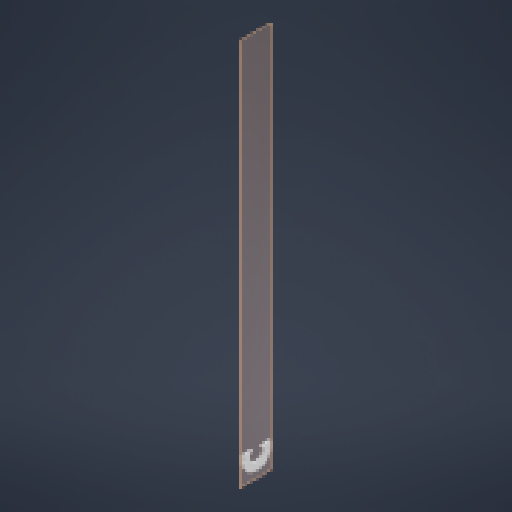
# Autodesk Inventor part: DropBarJoint
Saved by Autodesk Inventor 2024.1 (Build 281209000, 209)
## iProperties
Created: 2023-10-25
Part Number: DropBarJoint
Material: Generic
Document SubType Name: Modeling
Designer: Brandon
Density: 1 g/cm^3
Appearance: Default
Author: Brandon
Autodesk Inventor part; units mm, degrees
ref_plane "YZ Plane" through (0, 0, 0) normal (1, 0, 0) x (0, 1, 0)
ref_plane "XZ Plane" through (0, 0, 0) normal (0, 1, 0) x (-1, 0, 0)
ref_plane "XY Plane" through (0, 0, 0) normal (0, 0, 1) x (1, 0, 0)
ref_plane "Work Plane1" through (-214.9581, 261.0384, -210.6802) normal (1, 0, 0) x (0, 1, 0)
sketch "Sketch1" plane through (-214.9581, 261.0384, -210.6802) normal (1, 0, 0) x (0, 1, 0)
  arc A0 (-304.8, -19.05) -> (-298.45, -25.4) centre (-298.45, -19.05) ccw projected
  line L0 (-298.45, -25.4) -> (304.8, -25.4) projected
  line L1 (304.8, -25.4) -> (304.8, 25.4) projected
  line L2 (304.8, 25.4) -> (-298.45, 25.4) projected
  arc A1 (-298.45, 25.4) -> (-304.8, 19.05) centre (-298.45, 19.05) ccw projected
  line L3 (-304.8, 19.05) -> (-304.8, 17.2126) projected
  arc A2 (-304.8, 17.2126) -> (-297.523, 10.9306) centre (-298.45, 17.2126) ccw projected
  arc A3 (-297.523, -10.9306) -> (-297.523, 10.9306) centre (-295.91, 0) ccw projected
  arc A4 (-297.523, -10.9306) -> (-304.8, -17.2126) centre (-298.45, -17.2126) ccw projected
  line L4 (-304.8, -17.2126) -> (-304.8, -19.05) projected
  circle A5 centre (-295.91, 17.78) radius 2 projected
  circle A6 centre (-295.91, -17.78) radius 2 projected
  circle A7 centre (292.1, 12.7) radius 2 projected
  circle A8 centre (292.1, -12.7) radius 2 projected
  circle A9 centre (266.7, 12.7) radius 2 projected
  circle A10 centre (266.7, -12.7) radius 2 projected
  circle A11 centre (-295.91, 0) radius 11.049
  circle A12 centre (-295.91, 0) radius 25.4
  line L5 (-287.02, 23.7934) -> (-287.02, -23.7934)
  point P0 (-261.0384, 210.6802)
  point P1 (-287.02, 6.5611)
  point P2 (-287.02, -6.5611)
  point P3 (-297.523, -10.9306)
  dimension "d0" = 17.78
  constraints: 2 coincident, 2 end point, 2 point on circle, 1 centre point, 1 perpendicular, 1 tangent, 3 other
  measures "d0" distance from line of L5 L3.start
extrude "Extrusion1" add sketch "Sketch1" along normal blind 3 contours L4 A4 A3 L5 A12 A0 | A0 A12 A1 L3 A2 A11 A4 L4 | A12 L5 A3 A2 L3 A1
fillet "Fillet1" radius 6.35 4 edges at (-213.4581, -25.9816, -186.8868) (-213.4581, -25.9816, -217.2413) (-213.4581, -25.9816, -204.1191) (-213.4581, -25.9816, -234.4736)
body "Solid1"
